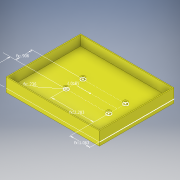
# Autodesk Inventor part: LargeCaseCaseBottomForPiZeroWV02
Saved by Autodesk Inventor 2019.4 (Build 234330000, 330)
## iProperties
Created: 2018-12-18
Part Number: LargeCaseCaseBottomForPiZeroWV02
Material: LCP Plastic
Document SubType Name: Modeling
Designer: steele
Density: 1.626 g/cm^3
Appearance: Yellow
PiZeroWLength: 2.559 in
PiZeroWWidth: 1.181 in
CaseLength: 3.150 in
CaseWidth: 1.772 in
CaseHeight: 0.515 in
PiZeroWMountingHole: 0.108 in
CaseWallThickness: 0.050 in
CaseFloorThickness: 0.200 in
PiZeroMoutingHolesLength: 2.283 in
PiZeroMountingHolesWidth: 0.906 in
PiZeroHoleSupport: 0.236 in
PiZeroWHoleHeight: 0.100 in
PiRibbonCableWidth: 0.787 in
PiRibbonCableThickness: 0.197 in
HdmiCenter: 0.748 in
MiniUsbCenter: 1.630 in
PowerCenter: 2.126 in
HdmiWidth: 1.102 in
MiniUsbWidth: 0.709 in
PowerWidth: 0.787 in
EndOfCaseToStartOfPiZero: 0.295 in
EyepieceOutsideDiameter: 1.250 in
EyepieceWallThickness: 0.075 in
EyepieceInnerDiameter: 1.100 in
PiRibbonCableHeightFromTp: 0.350 in
NutHeightPlusOffset: 0.073 in
NutWidthPlusOffset: 0.198 in
Author: steele
Autodesk Inventor part; units mm, degrees
ref_plane "YZ Plane" through (0, 0, 0) normal (1, 0, 0) x (0, 1, 0)
ref_plane "XZ Plane" through (0, 0, 0) normal (0, 1, 0) x (-1, 0, 0)
ref_plane "XY Plane" through (0, 0, 0) normal (0, 0, 1) x (1, 0, 0)
sketch "Sketch1" plane through (0, 0, 0) normal (0, 1, 0) x (-1, 0, 0)
  line L0 (63.5, 50.8) -> (-63.5, 50.8)
  line L1 (-63.5, 50.8) -> (-63.5, -50.8)
  line L2 (-63.5, -50.8) -> (63.5, -50.8)
  line L3 (63.5, -50.8) -> (63.5, 50.8)
  line L4 (63.5, 50.8) -> (-63.5, -50.8) construction
  line L5 (-63.5, 50.8) -> (63.5, -50.8) construction
  point P0 (0, 0)
  dimension "d0" = 127
  dimension "d1" = 101.6
  constraints: 12 end point, 2 midpoint, 2 parallel, 1 horizontal, 1 perpendicular
  measures "d0" distance of L1.end L2.end
  measures "d1" distance of L2.end L0.start
extrude "Extrusion1" add sketch "Sketch1" against normal blind 5.08
sketch "Sketch26" plane through (0, 0, 0) normal (0, 1, 0) x (1, 0, 0)
  line L0 (-21.5002, -11.0998) -> (36.4998, -11.0998) construction
  line L1 (36.4998, -11.0998) -> (36.4998, 11.9002) construction
  line L2 (36.4998, 11.9002) -> (-21.5002, 11.9002) construction
  line L3 (-21.5002, 11.9002) -> (-21.5002, -11.0998) construction
  line L4 (-63.5, -50.8) -> (63.5, -50.8) construction
  line L5 (63.5, -50.8) -> (-63.5, -50.8) construction
  circle A0 centre (-21.5002, -11.0998) radius 3
  circle A1 centre (-21.5002, 11.9002) radius 3
  circle A2 centre (36.4998, 11.9002) radius 3
  circle A3 centre (36.4998, -11.0998) radius 3
  line L6 (63.5, -50.8) -> (63.5, 50.8) projected
  line L7 (-21.5002, 0.4002) -> (36.4998, 0.4002) construction
  point P0 (0, 0)
  dimension "d173" = 58
  dimension "d174" = 23
  dimension "d175" = 39.7002
  dimension "d176" = 6
  dimension "d190" = 27.0002
  dimension "piZeroCenterLine" = 0.4002
  constraints: 10 end point, 4 centre point, 4 coincident, 3 equal radius, 2 midpoint, 2 parallel, 1 horizontal, 1 perpendicular
  measures "d173" distance of L0.start L0.end
  measures "d174" distance of L2.end L0.start
  measures "d175" distance between parallel lines of L4 L0
  measures "d176" diameter of A0
  measures "d190" distance between parallel lines of L6 L1
  measures "piZeroCenterLine" distance from line of point (0, 0) L7
extrude "Extrusion12" add sketch "Sketch26" along normal blind 2.54
sketch "Sketch27" plane through (0, -5.08, 0) normal (0, -1, 0) x (1, 0, 0)
  circle A0 centre (-21.5002, 11.0998) radius 3 projected
  circle A1 centre (-21.5002, -11.9002) radius 3 projected
  circle A2 centre (36.4998, -11.9002) radius 3 projected
  circle A3 centre (36.4998, 11.0998) radius 3 projected
  point P0 (0, 0)
  constraints: 4 coincident
hole "Hole17" at (-21.5002, -5.08, 11.0998) at (36.4998, -5.08, 11.0998) at (36.4998, -5.08, -11.9002) at (-21.5002, -5.08, -11.9002) direction (0, 1, 0) diameter 2.4384 end through all counterbore diameter 3.2639 counterbore depth 3.9878
sketch "Sketch28" plane through (0, 0, 0) normal (0, 1, 0) x (1, 0, 0)
  line L0 (63.5, -50.8) -> (-63.5, -50.8) projected
  line L1 (63.5, 50.8) -> (63.5, -50.8) projected
  line L2 (-63.5, -50.8) -> (63.5, -50.8)
  line L3 (63.5, -50.8) -> (63.5, 50.8)
  line L4 (63.5, 50.8) -> (-63.5, 50.8)
  line L5 (-63.5, 50.8) -> (-63.5, -50.8)
  line L6 (-62.23, -49.53) -> (62.23, -49.53)
  line L7 (62.23, -49.53) -> (62.23, 49.53)
  line L8 (62.23, 49.53) -> (-62.23, 49.53)
  line L9 (-62.23, 49.53) -> (-62.23, -49.53)
  line L10 (-62.23, -49.53) -> (62.23, 49.53) construction
  line L11 (62.23, -49.53) -> (-62.23, 49.53) construction
  point P0 (0, 0)
  dimension "d186" = 1.27
  dimension "d187" = 1.27
  constraints: 20 end point, 4 parallel, 2 horizontal, 2 midpoint, 2 perpendicular
  measures "d186" distance between parallel lines of L6 L0
  measures "d187" distance between parallel lines of L5 L9
extrude "Extrusion13" add sketch "Sketch28" along normal blind 13.08
sketch "Sketch22" plane through (0, -5.08, 0) normal (0, -1, 0) x (1, 0, 0)
  point P0 (34.92, -17.42)
  point P1 (34.92, 17.42)
  point P2 (-34.92, 17.42)
  point P3 (-34.92, -17.42)
equation "\"d0\" = LargeCaseLength"
equation "\"d1\" = LargeCaseWidth"
equation "\"d2\" = CaseFloorThickness"
equation "\"d173\" = PiZeroMoutingHolesLength"
equation "\"d174\" = PiZeroMountingHolesWidth"
equation "\"d175\" = PiZeroHolesDistanceFromSideWall"
equation "\"d176\" = PiZeroHoleSupport"
equation "\"d190\" = PiZeroHolesDistanceFromBottomWall"
equation "\"d177\" = PiZeroWHoleHeight"
equation "\"d186\" = CaseWallThickness"
equation "\"d187\" = CaseWallThickness"
equation "\"d188\" = CaseHeight"
equation "\"PiZeroWLength\" = 65"
equation "\"PiZeroWWidth\" = 30"
equation "\"CaseLength\" = PiZeroWLength + 2 * EndOfCaseToStartOfPiZero"
equation "\"CaseWidth\" = PiZeroWWidth + 2 * EndOfCaseToStartOfPiZero"
equation "\"PiZeroWMountingHole\" = 2.75"
equation "\"CaseWallThickness\" = 1.27"
equation "\"CaseFloorThickness\" = 5.08"
equation "\"PiZeroMoutingHolesLength\" = 58"
equation "\"PiZeroMountingHolesWidth\" = 23"
equation "\"PiZeroHoleSupport\" = 6"
equation "\"PiZeroWHoleHeight\" = 2.54"
equation "\"PiRibbonCableWidth\" = 20"
equation "\"PiRibbonCableThickness\" = 5"
equation "\"HdmiCenter\" = 19"
equation "\"MiniUsbCenter\" = 41.4"
equation "\"PowerCenter\" = 54"
equation "\"HdmiWidth\" = 28"
equation "\"MiniUsbWidth\" = 18"
equation "\"PowerWidth\" = 20"
equation "\"EndOfCaseToStartOfPiZero\" = 7.5"
equation "\"EyepieceOutsideDiameter\" = 31.75"
equation "\"EyepieceWallThickness\" = 1.905"
equation "\"EyepieceInnerDiameter\" = EyepieceOutsideDiameter - 2 * EyepieceWallThickness"
equation "\"HeightOfConnectorHolesAboveBottom\" = 6"
equation "\"HdmiHightAboveBottom\" = 6"
equation "\"MiniUsbHeightAboveBottom\" = 5"
equation "\"PowerHeightAboveBottom\" = 5"
equation "\"PiRibbonCableHeightFromTp\" = 8.89"
equation "\"NutHeightPlusOffset\" = 1.8415"
equation "\"NutWidthPlusOffset\" = 5.0165"
equation "\"LargeCaseWidth\" = 101.6"
equation "\"LargeCaseLength\" = 127"
equation "\"CameraHoleLength\" = 12.58"
equation "\"CameraHoleWidth\" = 21"
equation "\"PiZeroHolesDistanceFromSideWall\" = 39.7002"
equation "\"PiZeroHolesDistanceFromBottomWall\" = 27.0002"
equation "\"CaseHeight\" = 13.08"
body "Solid1"
